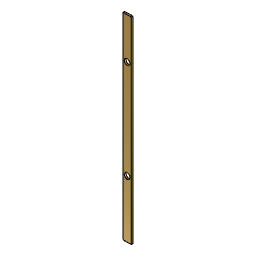
Mount Strip Left (Autodesk Fusion 360 design; units mm, degrees)
Autodesk Fusion 360 part; units mm, degrees
sketch "Sketch1" plane through (0, 0, 0) normal (0, 1, 0) x (1, 0, 0)
  line L0 (-5, -120) -> (5, -120)
  line L1 (5, -120) -> (5, 120)
  line L2 (5, 120) -> (-5, 120)
  line L3 (-5, 120) -> (-5, -120)
  circle A0 centre (0, -70) radius 3.5
  circle A1 centre (0, 50) radius 3.5
  dimension "d1" = 240
  dimension "d3" = 7
  dimension "d4" = 7
  dimension "d5" = 120
  dimension "d6" = 120
  dimension "d7" = 50
  constraint horizontal L0
  constraint vertical L1
  constraint horizontal L2
  constraint vertical L3
  measures "d1" distance of L0.start L2.end
  measures "d3" diameter of A0
  measures "d4" diameter of A1
  measures "d5" distance of A0.centre A1.centre
  measures "d6" distance of origin L0
  measures "d7" distance of L0 A0.centre
extrude "Extrude1" add sketch "Sketch1" along normal blind 2
named bodies: "Strip"
